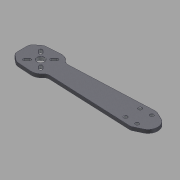
# Autodesk Inventor part: Arm
Saved by Autodesk Inventor 2011 SP2 (Build 150309200, 309)
## iProperties
Created: 2015-02-19
Part Number: Arm
Document SubType Name: Modeling
Designer: Greg Pavlik
Density: 1 g/cm^3
Author: Greg Pavlik
Autodesk Inventor part; units mm, degrees
ref_plane "YZ Plane" through (0, 0, 0) normal (1, 0, 0) x (0, 1, 0)
ref_plane "XZ Plane" through (0, 0, 0) normal (0, 1, 0) x (-1, 0, 0)
ref_plane "XY Plane" through (0, 0, 0) normal (0, 0, 1) x (1, 0, 0)
sketch "Sketch1" plane through (0, 0, 0) normal (0, 0, 1) x (1, 0, 0)
  line L0 (0, 0) -> (108, 0) construction
  arc A0 (111.5923, -7.7036) -> (111.5923, 7.7036) centre (108, 0) ccw
  line L1 (111.5923, 7.7036) -> (105.2612, 10.6558)
  line L2 (0, 4.0883) -> (0, -4.0883)
  line L3 (1.8874, 8.0013) -> (5.6994, 11.0335)
  line L4 (8.4632, 12.1083) -> (20.3247, 12.9377)
  line L5 (1.8874, -8.0013) -> (5.6994, -11.0335)
  line L6 (8.4632, -12.1083) -> (20.3247, -12.9377)
  arc A1 (27.5, 9.8365) -> (20.3247, 12.9377) centre (20.9177, 4.4584) ccw
  arc A2 (27.5, 9.8365) -> (31.5901, 8.0048) centre (31.372, 13) ccw
  line L7 (31.5901, 8.0048) -> (102.93, 11.1195)
  arc A3 (105.2612, 10.6558) -> (102.93, 11.1195) centre (103.1481, 6.1243) ccw
  line L8 (111.5923, -7.7036) -> (105.2612, -10.6558)
  arc A4 (20.3247, -12.9377) -> (27.5, -9.8365) centre (20.9177, -4.4584) ccw
  arc A5 (31.5901, -8.0048) -> (27.5, -9.8365) centre (31.372, -13) ccw
  line L9 (31.5901, -8.0048) -> (102.93, -11.1195)
  arc A6 (102.93, -11.1195) -> (105.2612, -10.6558) centre (103.1481, -6.1243) ccw
  arc A7 (5.6994, -11.0335) -> (8.4632, -12.1083) centre (8.812, -7.1205) ccw
  arc A8 (0, -4.0883) -> (1.8874, -8.0013) centre (5, -4.0883) ccw
  arc A9 (1.8874, 8.0013) -> (0, 4.0883) centre (5, 4.0883) ccw
  arc A10 (8.4632, 12.1083) -> (5.6994, 11.0335) centre (8.812, 7.1205) ccw
  line L10 (1.8858, 8) -> (31.372, 8) construction
  point P0 (0, 6.5)
  point P1 (0, -6.5)
  point P2 (6.9144, 12)
  point P3 (6.9144, -12)
  dimension "d0" = 13
  dimension "d1" = 77
  dimension "d2" = 8
  dimension "d3" = 8.5
  dimension "d4" = 5
  dimension "d5" = 5
  dimension "d6" = 27.5
  dimension "d7" = 24
  dimension "d8" = 5
  dimension "d9" = 108
  dimension "d10" = 8.5
  dimension "d11" = 50
  dimension "d12" = 5
  dimension "d13" = 8
  constraints: 24 point on circle, 22 end point, 15 tangent, 11 centre point, 11 symmetric about line, 8 point on line, 3 equal radius, 2 perpendicular, 1 coincident, 1 horizontal, 1 midpoint, 3 other
  measures "d0" distance of point (0, -6.5) point (0, 6.5)
  measures "d1" angle of L5 L3
  measures "d2" angle of L6 L4
  measures "d3" radius of A1
  measures "d4" radius of A2
  measures "d5" radius of A3
  measures "d6" distance from line of A1.start L2
  measures "d7" distance of point (6.914, -12) point (6.914, 12)
  measures "d8" radius of A7
  measures "d9" distance from line of L0.end L2
  measures "d10" radius of A0
  measures "d11" angle of L8 L1
  measures "d12" angle of L9 L7
  measures "d13" distance between parallel lines of L0 L10
extrude "Extrusion1" add sketch "Sketch1" along normal mid plane 3
sketch "Sketch2" plane through (0, 0, 1.5) normal (0, 0, 1) x (1, 0, 0)
  arc A0 (111.5923, -7.7036) -> (111.5923, 7.7036) centre (108, 0) ccw construction
  line L0 (0, -4.0883) -> (0, 4.0883) construction
  line L1 (108, 0) -> (0, 0) construction
  line L2 (95, 6.25) -> (105, 6.25)
  line L3 (105, 6.25) -> (105, -6.25)
  line L4 (105, -6.25) -> (95, -6.25)
  line L5 (95, -6.25) -> (95, 6.25)
  dimension "d16" = 12.5
  dimension "d17" = 10
  dimension "d18" = 95
  constraints: 10 end point, 4 coincident, 2 parallel, 2 perpendicular, 1 horizontal, 1 other
  measures "d16" distance between parallel lines of L4 L2
  measures "d17" distance between parallel lines of L3 L5
  measures "d18" distance between parallel lines of L0 L5
hole "Hole1" at (95, 6.25, 1.5) at (105, 6.25, 1.5) at (105, -6.25, 1.5) at (95, -6.25, 1.5) direction (0, 0, -1) diameter 3 end through all
sketch "Sketch3" plane through (0, 0, 1.5) normal (0, 0, 1) x (1, 0, 0)
  arc A0 (111.5923, -7.7036) -> (111.5923, 7.7036) centre (108, 0) ccw construction
  line L0 (0, -4.0883) -> (0, 4.0883) construction
  line L1 (0, 0) -> (108, 0) construction
  circle A1 centre (16, 0) radius 3.25
  line L2 (20.773, 4.773) -> (22.8943, 6.8943) construction
  circle A2 centre (16, 0) radius 9.75 construction
  circle A3 centre (16, 0) radius 6.75 construction
  arc A4 (23.7782, 6.0104) -> (22.0104, 7.7782) centre (22.8943, 6.8943) ccw
  arc A5 (19.8891, 5.6569) -> (21.6569, 3.8891) centre (20.773, 4.773) ccw
  line L3 (19.8891, 5.6569) -> (22.0104, 7.7782)
  line L4 (23.7782, 6.0104) -> (21.6569, 3.8891)
  arc A6 (9.9896, 7.7782) -> (8.2218, 6.0104) centre (9.1057, 6.8943) ccw
  arc A7 (10.3431, 3.8891) -> (12.1109, 5.6569) centre (11.227, 4.773) ccw
  line L5 (10.3431, 3.8891) -> (8.2218, 6.0104)
  line L6 (9.9896, 7.7782) -> (12.1109, 5.6569)
  arc A8 (8.2218, -6.0104) -> (9.9896, -7.7782) centre (9.1057, -6.8943) ccw
  arc A9 (12.1109, -5.6569) -> (10.3431, -3.8891) centre (11.227, -4.773) ccw
  line L7 (12.1109, -5.6569) -> (9.9896, -7.7782)
  line L8 (8.2218, -6.0104) -> (10.3431, -3.8891)
  arc A10 (22.0104, -7.7782) -> (23.7782, -6.0104) centre (22.8943, -6.8943) ccw
  arc A11 (21.6569, -3.8891) -> (19.8891, -5.6569) centre (20.773, -4.773) ccw
  line L9 (21.6569, -3.8891) -> (23.7782, -6.0104)
  line L10 (22.0104, -7.7782) -> (19.8891, -5.6569)
  dimension "d29" = 19.5
  dimension "d30" = 13.5
  dimension "d26" = 6.5
  dimension "d27" = 16
  dimension "d28" = 45
  dimension "d31" = 1.25
  dimension "d34" = 360
  constraints: 20 end point, 16 point on circle, 9 centre point, 4 coincident, 3 tangent, 2 parallel, 2 point on line, 1 perpendicular, 47 other
  measures "d26" diameter of A1
  measures "d27" distance from line of L0 A1.centre
  measures "d28" angle of L1 L2
  measures "d31" radius of A4
extrude "Extrusion2" cut sketch "Sketch3" against normal through all
chamfer "Chamfer1" distance 0.15 angle 45 34 edges at (19.8891, 3.8891, 1.5) (20.9497, 6.7175, 1.5) (23.7782, 7.7782, 1.5) (22.7175, 4.9497, 1.5) (12.75, 0, 1.5) (12.75, 0, -1.5) (22.7175, -4.9497, 1.5) (23.7782, -7.7782, 1.5) (20.9497, -6.7175, 1.5) (19.8891, -3.8891, 1.5) (22.7175, -4.9497, -1.5) (19.8891, -3.8891, -1.5) (20.9497, -6.7175, -1.5) (23.7782, -7.7782, -1.5) (8.2218, -7.7782, 1.5) (9.2825, -4.9497, 1.5) (12.1109, -3.8891, 1.5) (11.0503, -6.7175, 1.5) (12.1109, -3.8891, -1.5) (9.2825, -4.9497, -1.5) (8.2218, -7.7782, -1.5) (11.0503, -6.7175, -1.5) (9.2825, 4.9497, -1.5) (12.1109, 3.8891, -1.5) (11.0503, 6.7175, -1.5) (8.2218, 7.7782, -1.5) (12.1109, 3.8891, 1.5) (9.2825, 4.9497, 1.5) (8.2218, 7.7782, 1.5) (11.0503, 6.7175, 1.5) (23.7782, 7.7782, -1.5) (20.9497, 6.7175, -1.5) (19.8891, 3.8891, -1.5) (22.7175, 4.9497, -1.5)
chamfer "Chamfer2" distance 0.15 angle 45 8 edges at (95, -4.75, 1.5) (105, -4.75, 1.5) (95, 7.75, 1.5) (105, 7.75, 1.5) (95, -4.75, -1.5) (105, -4.75, -1.5) (95, 7.75, -1.5) (105, 7.75, -1.5)
chamfer "Chamfer3" distance 0.15 angle 45 40 edges at (108.4267, -9.1797, 1.5) (104.1236, -11.0282, 1.5) (67.26, -9.5621, 1.5) (29.3283, -8.4367, 1.5) (24.29, -12.2608, 1.5) (14.394, -12.523, 1.5) (6.9998, -11.7805, 1.5) (3.7934, -9.5174, 1.5) (0.4965, -6.2605, 1.5) (0, 0, 1.5) (0.4965, 6.2605, 1.5) (3.7934, 9.5174, 1.5) (6.9998, 11.7805, 1.5) (14.394, 12.523, 1.5) (24.29, 12.2608, 1.5) (29.3283, 8.4367, 1.5) (67.26, 9.5621, 1.5) (104.1236, 11.0282, 1.5) (108.4267, 9.1797, 1.5) (116.5, 0, 1.5) (108.4267, -9.1797, -1.5) (116.5, 0, -1.5) (108.4267, 9.1797, -1.5) (104.1236, 11.0282, -1.5) (67.26, 9.5621, -1.5) (29.3283, 8.4367, -1.5) (24.29, 12.2608, -1.5) (14.394, 12.523, -1.5) (6.9998, 11.7805, -1.5) (3.7934, 9.5174, -1.5) (0.4965, 6.2605, -1.5) (0, 0, -1.5) (0.4965, -6.2605, -1.5) (3.7934, -9.5174, -1.5) (6.9998, -11.7805, -1.5) (14.394, -12.523, -1.5) (24.29, -12.2608, -1.5) (29.3283, -8.4367, -1.5) (67.26, -9.5621, -1.5) (104.1236, -11.0282, -1.5)
body "Solid1"
